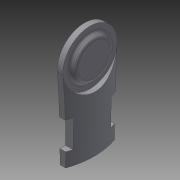
# Autodesk Inventor part: mid_curveUhorn
Saved by Autodesk Inventor 2014 (Build 180170000, 170)
## iProperties
Created: 2014-04-24
Part Number: mid_curveUhorn
Material: Generic
Document SubType Name: Modeling
Designer: t_emanb
Density: 1 g/cm^3
Appearance: Default
Author: t_emanb
Autodesk Inventor part; units mm, degrees
ref_plane "YZ Plane" through (0, 0, 0) normal (1, 0, 0) x (0, 1, 0)
ref_plane "XZ Plane" through (0, 0, 0) normal (0, 1, 0) x (-1, 0, 0)
sketch "Sketch1" plane through (0, 0, 0) normal (1, 0, 0) x (0, 1, 0)
  line L0 (-152.4, -22.225) -> (0, -22.225) construction
  line L1 (0, -22.225) -> (0, 22.225) construction
  line L2 (0, 22.225) -> (-152.4, 22.225) construction
  line L3 (-152.4, 22.225) -> (-152.4, -22.225) construction
  line L4 (-152.4, 0) -> (0, 0) construction
  arc A0 (-152.4, 22.225) -> (-152.4, -22.225) centre (-152.4, 0) ccw construction
  arc A1 (0, -22.225) -> (0, 22.225) centre (0, 0) ccw construction
  circle A2 centre (-152.4, 0) radius 2.95 construction
  circle A3 centre (0, 0) radius 2.95 construction
  arc A4 (-1.8103, -24.6987) -> (-1.8103, 24.6987) centre (0, 0) ccw
  line L5 (-76.2, 22.225) -> (-76.2, -22.225)
  line L6 (-35.56, 0) -> (-35.56, 22.225) construction
  line L7 (-76.2, 22.225) -> (-35.56, 22.225) construction
  line L8 (-35.56, 22.225) -> (-1.8103, 24.6987) construction
  spline S0 degree 2 poles (-76.2, 22.225) (-35.56, 22.225) (-1.8103, 24.6987) knots 1 1 1 2 2 2
  line L9 (-35.56, 0) -> (-35.56, -22.225) construction
  line L10 (-76.2, -22.225) -> (-35.56, -22.225) construction
  line L11 (-35.56, -22.225) -> (-1.8103, -24.6987) construction
  spline S1 degree 2 poles (-76.2, -22.225) (-35.56, -22.225) (-1.8103, -24.6987) knots 1 1 1 2 2 2
  dimension "d0" = 152.4
  dimension "d1" = 44.45
  dimension "d2" = 5.9
  dimension "d3" = 2.54
  dimension "d4" = 40.64
  constraints: 16 end point, 8 coincident, 6 point on circle, 5 centre point, 4 midpoint, 3 parallel, 3 symmetric about line, 2 horizontal, 1 equal radius, 1 perpendicular, 1 point on line, 1 tangent, 6 other
  measures "d0" distance of L2.end L1.end
  measures "d1" distance of L2.end L0.start
  measures "d2" diameter of A2
  measures "d3" radial gap between concentric circles of A4 A1
  measures "d4" distance between parallel lines of L5 L6
extrude "Extrusion1" add sketch "Sketch1" along normal blind 5.08
sketch "Sketch2" plane through (5.08, 0, 0) normal (1, 0, 0) x (0, 0, -1)
  arc A0 (24.6987, -1.8103) -> (-24.6987, -1.8103) centre (0, 0) ccw projected
  circle A1 centre (0, 0) radius 24.765
  line L0 (24.765, 0) -> (-24.765, 0)
  constraints: 4 point on circle, 2 coincident, 2 end point, 1 centre point, 1 concentric, 1 horizontal, 1 midpoint
ref_plane "Work Plane1" through (5.08, 0, -24.765) normal (0, 1, 0) x (0, 0, 1)
sketch "Sketch3" plane through (5.08, 0, -24.765) normal (0, 1, 0) x (0, 0, 1)
  line L0 (0, -5.08) -> (0, 0) projected
  line L1 (0.0663, -5.08) -> (49.4637, -5.08) projected
  line L2 (49.4637, -5.08) -> (49.4637, 0) projected
  line L3 (0.0663, 0) -> (49.4637, 0) projected
  line L4 (0.0663, -5.08) -> (0.0663, 0) projected
  arc A0 (49.4637, 0) -> (0.0663, 0) centre (24.765, -57.5021) ccw
  line L5 (24.765, -5.08) -> (24.765, 5.08) construction
  line L6 (49.4637, 0) -> (0.0663, 0)
  dimension "d8" = 10.16
  constraints: 4 end point, 3 point on circle, 1 centre point, 1 perpendicular
  measures "d8" distance of L5.start L5.end
sketch "Sketch4" plane through (0, -76.2, -22.225) normal (0, -1, 0) x (1, 0, 0)
  line L0 (5.08, 44.45) -> (5.08, 0) projected
  arc A0 (5.08, 0) -> (5.08, 44.45) centre (-57.8379, 22.225) ccw
  line L1 (0, 22.225) -> (8.89, 22.225) construction
  dimension "d9" = 8.89
  constraints: 3 point on circle, 2 end point, 1 centre point
  measures "d9" distance of L1.start L1.end
loft "Loft1" add profiles "Sketch4", "Sketch3" contours all / A0 L3
extrude "Extrusion2" cut sketch "Sketch2" along normal through all contours A1 A0 L0
sketch "Sketch6" plane through (0, -76.2, -22.225) normal (0, -1, 0) x (1, 0, 0)
  line L0 (0, 44.45) -> (0, 0) projected
  arc A0 (5.08, 0) -> (5.08, 44.45) centre (-57.8379, 22.225) ccw projected
  line L1 (1.778, 38.735) -> (5.588, 38.735)
  line L2 (5.588, 38.735) -> (5.588, 26.035)
  line L3 (5.588, 26.035) -> (1.778, 26.035)
  line L4 (1.778, 26.035) -> (1.778, 38.735)
  line L5 (0, 22.225) -> (8.89, 22.225) construction
  line L6 (1.778, 5.715) -> (5.588, 5.715)
  line L7 (5.588, 5.715) -> (5.588, 18.415)
  line L8 (5.588, 18.415) -> (1.778, 18.415)
  line L9 (1.778, 18.415) -> (1.778, 5.715)
  dimension "d19" = 12.7
  dimension "d20" = 3.81
  dimension "d21" = 1.778
  dimension "d63" = 7.62
  constraints: 18 end point, 4 symmetric about line, 2 parallel, 1 horizontal, 1 perpendicular, 1 point on circle
  measures "d19" distance of L1.end L2.end
  measures "d20" distance of L2.end L3.end
  measures "d21" distance between parallel lines of L0 L4
  measures "d63" distance between parallel lines of L3 L8
extrude "Extrusion4" cut sketch "Sketch6" against normal blind 12.7
sketch "Sketch8" plane through (0, 0, 0) normal (-1, 0, 0) x (0, 0, 1)
  line L0 (22.225, -76.2) -> (-22.225, -76.2) projected
  spline S0 degree 2 poles (24.6987, -1.8103) (22.225, -35.56) (22.225, -76.2) knots 0 0 0 1 1 1 projected
  arc A0 (24.6987, -1.8103) -> (-24.6987, -1.8103) centre (0, 0) ccw projected
  spline S1 degree 2 poles (-22.225, -76.2) (-22.225, -35.56) (-24.6987, -1.8103) knots 0 0 0 1 1 1 projected
  line L1 (-22.225, -76.2) -> (-24.765, -76.2)
  line L2 (-24.765, -76.2) -> (-24.765, 0)
  line L3 (22.225, -76.2) -> (24.765, -76.2)
  line L4 (24.765, -76.2) -> (24.765, 0)
  constraints: 8 end point, 2 point on circle, 2 tangent, 2 vertical, 1 collinear, 1 perpendicular, 2 other
extrude "Extrusion6" cut sketch "Sketch8" against normal through all contours S0 A0 L4 L3 | L1 L2 A0 S1
sketch "Sketch9" plane through (0, 0, 0) normal (-1, 0, 0) x (0, 0, 1)
  line L0 (22.225, -76.2) -> (-22.225, -76.2) projected
  spline S0 degree 2 poles (24.6987, -1.8103) (22.225, -35.56) (22.225, -76.2) knots 0 0 0 1 1 1 projected
  arc A0 (24.6987, -1.8103) -> (-24.6987, -1.8103) centre (0, 0) ccw projected
  spline S1 degree 2 poles (-22.225, -76.2) (-22.225, -35.56) (-24.6987, -1.8103) knots 0 0 0 1 1 1 projected
  line L1 (-22.2883, -63.373) -> (-17.2083, -63.373)
  line L2 (-17.2083, -63.373) -> (-17.2083, -38.1)
  line L3 (-17.2083, -38.1) -> (-22.8166, -38.1)
  line L4 (22.2883, -63.373) -> (17.2083, -63.373)
  line L5 (17.2083, -63.373) -> (17.2083, -38.1)
  line L6 (17.2083, -38.1) -> (22.8166, -38.1)
  dimension "d38" = 5.08
  dimension "d39" = 5.08
  dimension "d40" = 25.273
  dimension "d41" = 38.1
  constraints: 12 end point, 4 parallel, 2 collinear, 2 perpendicular, 6 other
  measures "d38" distance of L1.start L1.end
  measures "d39" distance of L4.start L4.end
  measures "d40" distance of L1.end L2.end
  measures "d41" distance from line of A0.centre L3
extrude "Extrusion7" cut sketch "Sketch9" against normal through all contours L4 L5 L6 S0 | S1 L3 L2 L1
sketch "Sketch10" plane through (5.08, 0, 0) normal (1, 0, 0) x (0, 0, -1)
  arc A0 (-24.6085, -2.7797) -> (24.6085, -2.7797) centre (0, 0) ccw projected
  line L0 (0, 0) -> (0, 12) construction
  circle A1 centre (0, 0) radius 4.1275 construction
  arc A2 (2, 10.2354) -> (-2, 10.2354) centre (0, 9.9843) ccw
  line L1 (0, 0) -> (-2.9186, 2.9186) construction
  line L2 (0, 0) -> (-12, 0) construction
  line L3 (-2.9186, 2.9186) -> (-2, 10.2354)
  line L4 (0, 0) -> (2.9186, 2.9186) construction
  line L5 (2.9186, 2.9186) -> (2, 10.2354)
  line L6 (-2.9186, 2.9186) -> (-10.2354, 2)
  arc A3 (-10.2354, 2) -> (-10.2354, -2) centre (-9.9843, 0) ccw
  line L7 (-2.9186, -2.9186) -> (-10.2354, -2)
  line L8 (-2.9186, -2.9186) -> (-2, -10.2354)
  arc A4 (-2, -10.2354) -> (2, -10.2354) centre (0, -9.9843) ccw
  line L9 (2.9186, -2.9186) -> (2, -10.2354)
  line L10 (2.9186, 2.9186) -> (10.2354, 2)
  arc A5 (10.2354, -2) -> (10.2354, 2) centre (9.9843, 0) ccw
  line L11 (2.9186, -2.9186) -> (10.2354, -2)
  dimension "d45" = 8.255
  dimension "d44" = 12
  dimension "d46" = 45
  dimension "d47" = 4
  constraints: 24 end point, 13 symmetric about line, 9 point on circle, 4 centre point, 2 coincident, 2 perpendicular, 1 point on line, 1 tangent, 1 vertical, 6 other
  measures "d44" distance of L0.start L0.end
  measures "d46" angle of L1 L2
  measures "d47" distance of L5.end L3.end
extrude "Extrusion8" cut sketch "Sketch10" against normal through all
sketch "Sketch11" plane through (5.08, 0, 0) normal (1, 0, 0) x (0, 0, -1)
  arc A0 (-24.6085, -2.7797) -> (24.6085, -2.7797) centre (0, 0) ccw projected
  circle A1 centre (0, 0) radius 17.78
  dimension "d50" = 35.56
  constraints: 1 centre point, 1 coincident
  measures "d50" diameter of A1
extrude "Extrusion9" add sketch "Sketch11" along normal blind 3.81
sketch "Sketch14" plane through (5.08, 0, 0) normal (-1, 0, 0) x (0, 0, 1)
  circle A0 centre (0, 0) radius 1.016
  circle A1 centre (0, 0) radius 2.794
  line L0 (-10.2354, -2) -> (-2.9186, -2.9186) projected
  line L1 (-2.9186, -2.9186) -> (-2, -10.2354) projected
  arc A2 (-2, -10.2354) -> (2, -10.2354) centre (0, -9.9843) ccw projected
  line L2 (2, -10.2354) -> (2.9186, -2.9186) projected
  line L3 (2.9186, -2.9186) -> (10.2354, -2) projected
  arc A3 (10.2354, -2) -> (10.2354, 2) centre (9.9843, 0) ccw projected
  line L4 (10.2354, 2) -> (2.9186, 2.9186) projected
  line L5 (2.9186, 2.9186) -> (2, 10.2354) projected
  arc A4 (2, 10.2354) -> (-2, 10.2354) centre (0, 9.9843) ccw projected
  line L6 (-2, 10.2354) -> (-2.9186, 2.9186) projected
  line L7 (-2.9186, 2.9186) -> (-10.2354, 2) projected
  arc A5 (-10.2354, 2) -> (-10.2354, -2) centre (-9.9843, 0) ccw projected
  dimension "d59" = 5.588
  constraints: 2 centre point, 1 coincident
  measures "d59" diameter of A1
extrude "Extrusion12" cut sketch "Sketch14" against normal blind 1.016 contours A0 | A1
fillet "Fillet1" radius 3.175 2 edges at (8.89, 0, 17.78) (5.08, 0, 17.78)
fillet "Fillet2" radius 1.27 8 edges at (3.683, -63.5, -3.81) (3.683, -76.2, -3.81) (3.683, -76.2, -16.51) (3.683, -63.5, -16.51) (3.683, -76.2, 3.81) (3.683, -76.2, 16.51) (3.683, -63.5, 16.51) (3.683, -63.5, 3.81)
body "Solid1"
